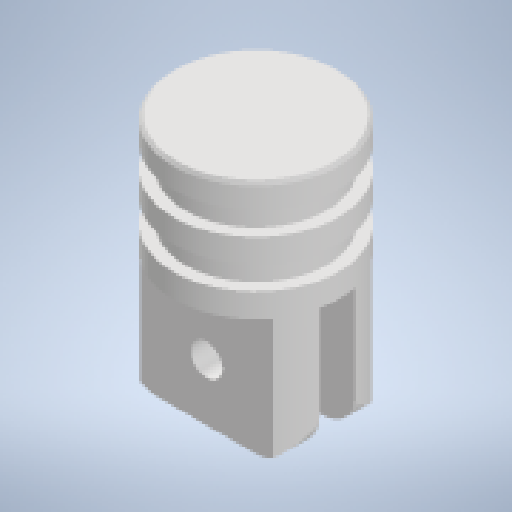
# Autodesk Inventor part: Piston Head
Saved by Autodesk Inventor 2023 (Build 270158000, 158)
## iProperties
Created: 2022-10-26
Part Number: Piston Head
Material: Generic
Document SubType Name: Modeling
Designer: tommy
Density: 1 g/cm^3
Appearance: Default
Author: tommy
Autodesk Inventor part; units mm, degrees
ref_plane "YZ Plane" through (0, 0, 0) normal (1, 0, 0) x (0, 1, 0)
ref_plane "XZ Plane" through (0, 0, 0) normal (0, 1, 0) x (-1, 0, 0)
ref_plane "XY Plane" through (0, 0, 0) normal (0, 0, 1) x (1, 0, 0)
sketch "Sketch5" plane through (0, 0, 0) normal (1, 0, 0) x (0, 1, 0)
  line L0 (15.875, -16.6688) -> (15.875, -14.2875)
  line L1 (15.875, -14.2875) -> (20.6375, -14.2875)
  line L2 (20.6375, -14.2875) -> (20.6375, -16.6688)
  line L3 (20.6375, -16.6688) -> (25.4, -16.6688)
  line L4 (25.4, -16.6688) -> (25.4, -14.2875)
  line L5 (25.4, -14.2875) -> (30.1625, -14.2875)
  line L6 (30.1625, -14.2875) -> (30.1625, -16.6688)
  line L7 (30.1625, -16.6688) -> (34.925, -16.6688)
  line L8 (34.925, -16.6688) -> (34.925, 0)
  line L9 (15.875, -16.6688) -> (11.0998, -16.6688)
  line L10 (34.925, 0) -> (11.0998, 0)
  line L11 (11.0998, -16.6688) -> (11.0998, 0)
  dimension "d15" = 2.3813
  dimension "d16" = 4.7625
  dimension "d17" = 4.7625
  dimension "d18" = 4.7625
  dimension "d19" = 4.7625
  dimension "d38" = 4.7752
  constraints: 24 end point, 4 point on line, 3 perpendicular, 2 vertical, 1 horizontal, 1 parallel
  measures "d15" distance of L0.start L0.end
  measures "d16" distance of L0.end L1.end
  measures "d17" distance of L2.end L3.end
  measures "d18" distance of L4.end L5.end
  measures "d19" distance of L6.end L7.end
  measures "d38" distance of L0.start L9.end
revolve "Revolution1" add sketch "Sketch5" angle 360 about axis through (0, 34.925, 0) along (0, -1, 0)
chamfer "Chamfer1" distance 0.635 angle 45 1 edges at (0, 34.925, 16.6688)
sketch "Sketch10" plane through (0, 11.0998, 0) normal (0, -1, 0) x (1, 0, 0)
  circle A0 centre (0, 0) radius 16.6687
  circle A1 centre (0, 0) radius 16.6687 projected
  line L0 (16.2822, 3.5687) -> (-16.2822, 3.5687)
  line L1 (16.2822, -3.5687) -> (-16.2822, -3.5687)
  line L2 (13.3965, 9.9187) -> (-13.3965, 9.9187)
  line L3 (13.3965, -9.9187) -> (-13.3965, -9.9187)
  point P0 (-13.3965, -9.9187)
  point P1 (13.3965, -9.9187)
  point P2 (16.2822, -3.5687)
  point P3 (-16.2822, -3.5687)
  constraints: 8 end point, 8 point on circle, 2 horizontal, 1 centre point, 1 coincident
extrude "Extrusion6" add sketch "Sketch10" along normal blind 25.4 contours L0 A0 L2 | A0 L3 L1
sketch "Sketch12" plane through (13.3965, 11.0998, -9.9187) normal (0, 0, -1) x (-1, 0, 0)
  line L0 (-2.8857, -25.4) -> (29.6788, -25.4) projected
  circle A0 centre (13.3965, -13.97) radius 3.175
  line L1 (29.6788, 0) -> (29.6788, -25.4) projected
  line L2 (23.3288, -25.4) -> (13.3965, -25.4)
  line L3 (-2.8857, 0) -> (-2.8857, -25.4) projected
  line L4 (-2.8857, -12.7) -> (-2.8857, -19.05)
  line L5 (13.3965, -25.4) -> (3.4643, -25.4)
  arc A1 (-2.8857, -19.05) -> (3.4643, -25.4) centre (3.4643, -19.05) ccw
  line L6 (29.6788, -12.7) -> (29.6788, -19.05)
  arc A2 (23.3288, -25.4) -> (29.6788, -19.05) centre (23.3288, -19.05) ccw
  line L7 (29.6788, -12.7) -> (35.365, -12.7)
  line L8 (35.365, -12.7) -> (34.5299, -34.8796)
  line L9 (34.5299, -34.8796) -> (-9.3415, -34.8796)
  line L10 (-9.3415, -34.8796) -> (-9.3415, -12.7)
  line L11 (-9.3415, -12.7) -> (-2.8857, -12.7)
  point P0 (13.3965, -11.0998)
  point P1 (3.4643, -25.4)
  dimension "d68" = 6.35
  dimension "d69" = 6.35
  dimension "d70" = 6.35
  constraints: 18 end point, 5 point on line, 4 point on circle, 4 tangent, 3 centre point, 3 collinear, 3 midpoint, 2 perpendicular, 1 horizontal, 1 parallel
  measures "d68" diameter of A0
  measures "d69" radius of A1
  measures "d70" radius of A2
extrude "Extrusion7" cut sketch "Sketch12" against normal blind 25.4
sketch "Sketch13" plane through (-16.2822, 11.0998, -3.5687) normal (0, 0, 1) x (1, 0, 0)
  line L0 (0, 0) -> (32.5645, 0) projected
  line L1 (-0.3865, 4.7752) -> (-0.3865, 0) projected
  arc A0 (32.5645, 0) -> (-0.3865, 0) centre (16.089, -41.6307) ccw
  line L2 (32.5645, 0) -> (32.5645, -4.0672)
  line L3 (32.5645, 0) -> (32.5645, -19.05) projected
  line L4 (32.5645, -4.0672) -> (-0.3865, -4.0672)
  line L5 (-0.3865, -4.0672) -> (-0.3865, 0)
  line L6 (32.5645, 0) -> (32.5645, -4.0672)
  point P0 (16.2822, -11.0998)
  constraints: 8 end point, 2 point on circle, 2 point on line, 1 centre point, 1 horizontal, 1 parallel, 1 perpendicular
extrude "Extrusion8" cut sketch "Sketch13" along normal blind 7.1374
body "Solid3"
